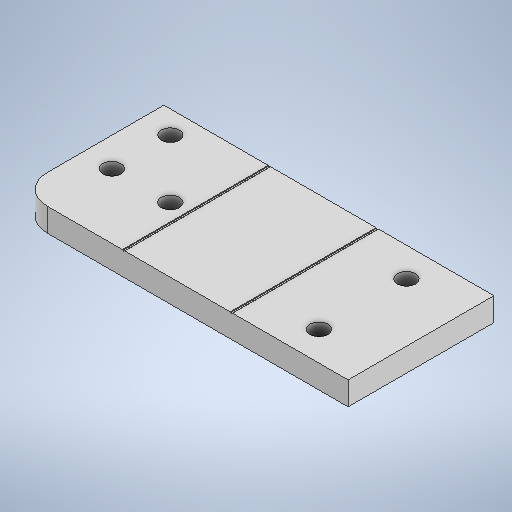
# Autodesk Inventor part: GVS_Plate
Saved by Autodesk Inventor 2025 (Build 290162000, 162)
## iProperties
Created: 2025-05-19
Part Number: GVS_Plate
Material: Generic
Document SubType Name: Modeling
Designer: mumin
Density: 1 g/cm^3
Appearance: Default
Author: mumin
Autodesk Inventor part; units mm, degrees
ref_plane "YZ Plane" through (0, 0, 0) normal (1, 0, 0) x (0, 1, 0)
ref_plane "XZ Plane" through (0, 0, 0) normal (0, 1, 0) x (-1, 0, 0)
ref_plane "XY Plane" through (0, 0, 0) normal (0, 0, 1) x (1, 0, 0)
sketch "Sketch1" plane through (0, 0, 0) normal (0, 1, 0) x (-1, 0, 0)
  line L0 (10.5834, 13.2197) -> (-45.9966, 13.2197)
  line L1 (-45.9966, 13.2197) -> (-45.9966, -11.7803)
  line L2 (-45.9966, -11.7803) -> (10.5834, -11.7803)
  line L3 (10.5834, -11.7803) -> (10.5834, 13.2197)
  circle A0 centre (5.5834, -7.8803) radius 1.55
  circle A1 centre (5.5834, 2.1197) radius 1.55
  circle A2 centre (-4.4166, 2.1197) radius 1.55
  circle A3 centre (-35.9966, 8.2197) radius 1.55
  circle A4 centre (-35.9966, -6.7803) radius 1.55
  point P0 (0, 0)
  dimension "d0" = 3.1
  dimension "d1" = 3.9
  dimension "d4" = 10
  dimension "d11" = 10
  dimension "d16" = 25
  dimension "d17" = 5
  dimension "d18" = 56.58
  dimension "d19" = 3.1
  dimension "d20" = 10
  dimension "d23" = 15
  dimension "d28" = 5
  constraints: 8 end point, 5 centre point, 2 horizontal, 2 parallel, 2 vertical, 1 perpendicular, 6 other
  measures "d0" diameter of A0
  measures "d1" distance from line of L2 A0.centre
  measures "d4" distance of A0.centre A1.centre
  measures "d11" distance of A1.centre A2.centre
  measures "d16" distance of L2.end L0.start
  measures "d17" distance from line of L3 A0.centre
  measures "d18" distance of L0.start L0.end
  measures "d19" diameter of A3
  measures "d20" distance from line of L1 A3.centre
  measures "d23" distance of A3.centre A4.centre
  measures "d28" distance from line of A3.centre L0
extrude "Extrusion1" add sketch "Sketch1" along normal mid plane 4
sketch "Sketch2" plane through (45.9966, 2, -11.7803) normal (0, 0, -1) x (-1, 0, 0)
  arc A0 (38.37, 0) -> (38.62, 0) centre (38.495, 0) ccw
  line L0 (0, 0) -> (56.58, 0) projected
  line L1 (56.58, -4) -> (56.58, 0) projected
  circle A1 centre (20, 0) radius 0.125
  line L2 (0, -4) -> (0, 0) projected
  point P0 (45.9966, -2)
  point P1 (56.58, -2)
  point P2 (20.125, 0)
  point P3 (19.875, 0)
  dimension "d31" = 0.25
  dimension "d34" = 18.085
  dimension "d35" = 0.25
  dimension "d36" = 20
  constraints: 4 point on line, 2 centre point, 2 point on circle, 1 midpoint
  measures "d31" diameter of A0
  measures "d34" horizontal distance of point (56.58, -2) A0.centre
  measures "d35" diameter of A1
  measures "d36" distance from line of L2 A1.centre
extrude "Extrusion2" cut sketch "Sketch2" against normal up to surface (25 mm away) contours L0 A0 | A1 L0 picked at (20, -0.0736)
fillet "Fillet1" radius 0.1 4 edges at (7.6266, 2, 0.7197) (7.3766, 2, 0.7197) (26.1216, 2, 0.7197) (25.8716, 2, 0.7197)
fillet "Fillet2" radius 5 1 edges at (-10.5834, 0, 13.2197)
body "Solid1"
